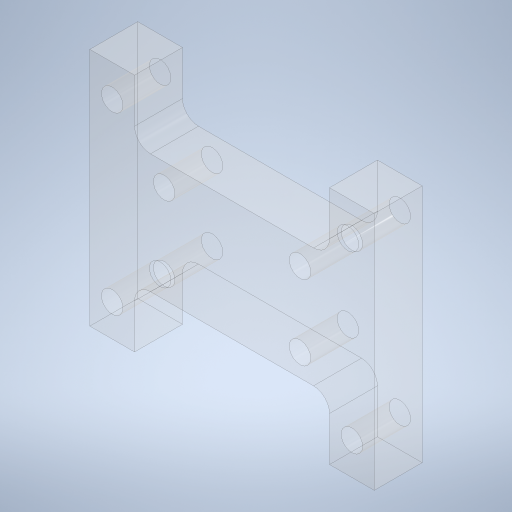
# Autodesk Inventor part: frame_arm_to_hand1
Saved by Autodesk Inventor 2024 (Build 280153000, 153)
## iProperties
Created: 2024-09-06
Part Number: frame_arm_to_hand1
Material: PMMA 플라스틱
Document SubType Name: Modeling
Designer: jmha0
Density: 1.188 g/cm^3
Appearance: 폴리카보네이트 - 선명
Mass: 9.71643 g
Surface Area: 43.5089 cm^2
Volume: 8.17881 cm^3
Author: jmha0
Autodesk Inventor part; units mm, degrees
ref_plane "YZ Plane" through (0, 0, 0) normal (1, 0, 0) x (0, 1, 0)
ref_plane "XZ Plane" through (0, 0, 0) normal (0, 1, 0) x (-1, 0, 0)
ref_plane "XY Plane" through (0, 0, 0) normal (0, 0, 1) x (1, 0, 0)
sketch "스케치1" plane through (0, 0, 0) normal (0, 0, 1) x (1, 0, 0)
  line L0 (22.3806, -23.2436) -> (22.3806, 15.7564)
  arc A0 (20.3806, -26.2436) -> (22.3806, -24.2436) centre (20.3806, -24.2436) ccw
  line L1 (22.3806, -24.2436) -> (22.3806, -22.8439)
  line L2 (18.7808, -26.2436) -> (20.3806, -26.2436)
  line L3 (0.9806, -26.2436) -> (19.3806, -26.2436)
  arc A1 (-2.0194, -24.2436) -> (-0.0194, -26.2436) centre (-0.0194, -24.2436) ccw
  line L4 (-0.0194, -26.2436) -> (1.5803, -26.2436)
  line L5 (-2.0194, -24.2436) -> (-2.0194, -22.8439)
  line L6 (-2.0194, 15.7564) -> (-2.0194, -23.2436)
  circle A2 centre (25.1806, -22.7436) radius 1.45
  circle A3 centre (18.6806, -29.0436) radius 1.45
  circle A4 centre (1.6806, -29.0436) radius 1.45
  circle A5 centre (-4.8194, -22.7436) radius 1.45
  line L7 (-7.6194, -18.7138) -> (27.9806, -18.7138)
  line L8 (-7.6194, -18.7138) -> (27.9806, -18.7138)
  arc A6 (-0.0194, -41.1839) -> (-2.0194, -43.1839) centre (-0.0194, -43.1839) ccw
  line L9 (-2.0194, -43.1839) -> (-2.0194, -44.5837)
  line L10 (1.5803, -41.1839) -> (-0.0194, -41.1839)
  line L11 (19.3806, -41.1839) -> (0.9806, -41.1839)
  arc A7 (22.3806, -43.1839) -> (20.3806, -41.1839) centre (20.3806, -43.1839) ccw
  line L12 (20.3806, -41.1839) -> (18.7808, -41.1839)
  line L13 (22.3806, -43.1839) -> (22.3806, -44.5837)
  circle A8 centre (-4.8194, -44.6839) radius 1.45
  circle A9 centre (1.6806, -38.3839) radius 1.45
  circle A10 centre (18.6806, -38.3839) radius 1.45
  circle A11 centre (25.1806, -44.6839) radius 1.45
  line L14 (27.9806, -48.7138) -> (-7.6194, -48.7138)
  line L15 (27.9806, -48.7138) -> (-7.6194, -48.7138)
  line L16 (-2.0194, -44.5837) -> (-2.0194, -48.7138)
  line L17 (22.3806, -44.5837) -> (22.3806, -48.7138)
  line L18 (10.1806, -18.7138) -> (10.1806, -33.7138)
  line L19 (-7.6194, -48.7138) -> (27.9806, -48.7138)
  line L20 (27.9806, -48.7138) -> (27.9806, -33.7138)
  line L21 (27.9806, -33.7138) -> (-7.6194, -33.7138)
  line L22 (-7.6194, -33.7138) -> (-7.6194, -48.7138)
  circle A12 centre (10.1806, -33.7138) radius 2.4281
  line L23 (-7.6194, -18.7138) -> (-7.6194, -34.6206)
  line L24 (27.9806, -18.7138) -> (27.9806, -33.7138)
  circle A13 centre (-4.8194, -22.7436) radius 1.35
  circle A14 centre (1.6806, -29.0436) radius 1.35
  circle A15 centre (18.6806, -29.0436) radius 1.35
  circle A16 centre (25.1806, -22.7436) radius 1.35
  circle A17 centre (18.6806, -38.3839) radius 1.35
  circle A18 centre (25.1806, -44.6839) radius 1.35
  circle A19 centre (1.6806, -38.3839) radius 1.35
  circle A20 centre (-4.8194, -44.6839) radius 1.35
  point P0 (0, 0)
  point P1 (-7.1939, 58.7329)
  point P2 (22.3806, -18.7138)
  point P3 (-2.0194, -18.7138)
  point P4 (27.9806, -25.8436)
  point P5 (-7.6194, -25.8436)
  point P6 (-2.0194, -44.1839)
  point P7 (-7.6194, -41.5839)
  point P8 (22.3806, -44.1839)
  point P9 (27.9806, -41.5839)
  point P10 (-2.0194, -18.7138)
  point P11 (22.3806, -18.7138)
  point P12 (10.1806, -48.7138)
  dimension "d11" = 30
  dimension "d12" = 15
  dimension "d13" = 15
  dimension "d14" = 2.7
  dimension "d15" = 2.7
  dimension "d16" = 2.7
  dimension "d17" = 2.7
  dimension "d18" = 2.7
  dimension "d19" = 2.7
  dimension "d20" = 2.7
  dimension "d21" = 2.7
  constraints: 50 end point, 21 centre point, 8 coincident, 8 point on circle, 4 point on line, 3 midpoint, 3 parallel, 3 perpendicular, 2 horizontal
  measures "d11" distance of point (10.181, -48.714) L18.start
  measures "d12" distance of L18.start L18.end
  measures "d13" distance of L20.end L19.end
  measures "d14" diameter of A13
  measures "d15" diameter of A14
  measures "d16" diameter of A15
  measures "d17" diameter of A16
  measures "d18" diameter of A17
  measures "d19" diameter of A18
  measures "d20" diameter of A19
  measures "d21" diameter of A20
extrude "돌출1" add sketch "스케치1" along normal blind 6 contours L0 L7 L24 L21 A12 L18 L3 L2 A0 L1 | L6 L5 A1 L4 L3 L18 A12 L21 L23 L7 | L20 L14 L17 L13 A7 L12 L11 L10 A6 L9 L16 L22 L21 A12 | A12 L21 L18 | L18 L21 A12 | A12 L21 | A2 | A3 | A4 | A5 | A8 | A9 | A10 | A11
